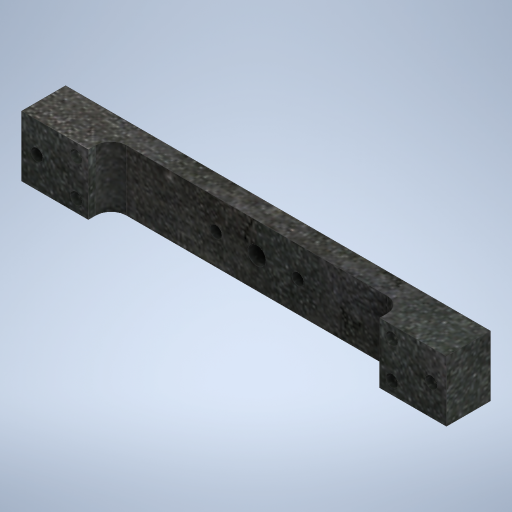
# Autodesk Inventor part: Uchwyt na ramę
Saved by Autodesk Inventor 2024 (Build 280153000, 153)
## iProperties
Created: 2024-04-14
Part Number: Uchwyt na ramę
Material: Steel
Document SubType Name: Sheet Metal
Designer: HP
Density: 7.85 g/cm^3
Sheet Metal Rule: Default
Appearance: Plate
Author: HP
Autodesk Inventor part; units mm, degrees
ref_plane "YZ Plane" through (0, 0, 0) normal (1, 0, 0) x (0, 1, 0)
ref_plane "XZ Plane" through (0, 0, 0) normal (0, 1, 0) x (-1, 0, 0)
ref_plane "XY Plane" through (0, 0, 0) normal (0, 0, 1) x (1, 0, 0)
sketch "Sketch1" plane through (0, 0, 0) normal (0, 0, 1) x (1, 0, 0)
  line L0 (-70, 10) -> (70, 10)
  line L1 (70, 10) -> (70, -10)
  line L2 (70, -10) -> (-70, -10)
  line L3 (-70, -10) -> (-70, 10)
  line L4 (-70, 10) -> (70, -10) construction
  line L5 (70, 10) -> (-70, -10) construction
  line L6 (0, 0) -> (-13.5, 0) construction
  line L7 (-13.5, 0) -> (13.5, 0) construction
  circle A0 centre (-13.5, 0) radius 2
  circle A1 centre (13.5, 0) radius 2
  circle A2 centre (0, 0) radius 3
  dimension "d0" = 140
  dimension "d1" = 20
  dimension "d2" = 13.5
  dimension "d3" = 27
  dimension "d4" = 4
  dimension "d5" = 4
  dimension "d6" = 6
  constraints: 16 end point, 3 centre point, 3 coincident, 2 horizontal, 2 midpoint, 2 parallel, 1 perpendicular, 1 point on line
  measures "d0" distance of L1.end L2.end
  measures "d1" distance of L0.end L1.end
  measures "d2" distance of L6.start L6.end
  measures "d3" distance of L6.end L7.end
  measures "d4" diameter of A0
  measures "d5" diameter of A1
  measures "d6" diameter of A2
extrude "Extrusion1" add sketch "Sketch1" along normal mid plane 7
sketch "Sketch2" plane through (-70, -10, 3.5) normal (0, -1, 0) x (1, 0, 0)
  line L0 (70, -3.5) -> (30, -3.5) construction
  line L1 (30, -3.5) -> (110, -3.5) construction
  line L2 (0, 0) -> (140, 0) projected
  line L3 (22, 5) -> (22, 7.5)
  line L4 (22, 7.5) -> (2, 7.5)
  line L5 (0, 5.5) -> (0, 0)
  line L6 (0, 0) -> (22, 0)
  line L7 (70, -9.525) -> (70, 0) construction
  line L8 (27, 0) -> (140, 0)
  arc A0 (22, 5) -> (27, 0) centre (27, 5) ccw
  line L9 (27, 0) -> (22, 0)
  line L10 (140, 0) -> (0, 0)
  line L11 (118, 5) -> (118, 7.5)
  line L12 (118, 7.5) -> (138, 7.5)
  line L13 (140, 5.5) -> (140, 0)
  arc A1 (113, 0) -> (118, 5) centre (113, 5) ccw
  line L14 (140, 5.5) -> (140, 7.5)
  line L15 (140, 7.5) -> (138, 7.5)
  line L16 (0, 5.5) -> (0, 7.5)
  line L17 (0, 7.5) -> (2, 7.5)
  point P0 (113, 0)
  dimension "d13" = 40
  dimension "d14" = 80
  dimension "d15" = 7.5
  dimension "d16" = 5
  constraints: 34 end point, 8 symmetric about line, 5 perpendicular, 4 point on circle, 4 point on line, 3 tangent, 2 centre point, 2 collinear, 2 horizontal, 2 vertical, 1 midpoint, 1 other
  measures "d13" distance of L0.start L0.end
  measures "d14" distance of L0.end L1.end
  measures "d15" distance of L6.end L3.end
  measures "d16" radius of A0
extrude "Extrusion2" add sketch "Sketch2" against normal blind 20
sketch "Sketch3" plane through (48, -10, 11) normal (0, 0, 1) x (1, 0, 0)
  line L0 (-48, 10) -> (12, 10) construction
  line L1 (12, 10) -> (17, 10) construction
  circle A0 centre (17, 10) radius 2
  line L2 (12, 10) -> (4, 10) construction
  line L3 (4, 10) -> (4, 4) construction
  line L4 (4, 4) -> (4, 16) construction
  circle A1 centre (4, 4) radius 2
  circle A2 centre (4, 16) radius 2
  line L5 (-48, 10) -> (-48, 19.9246) construction
  circle A3 centre (-113, 10) radius 2
  circle A4 centre (-100, 4) radius 2
  circle A5 centre (-100, 16) radius 2
  dimension "d20" = 60
  dimension "d21" = 5
  dimension "d22" = 4
  dimension "d23" = 8
  dimension "d24" = 6
  dimension "d25" = 12
  dimension "d26" = 4
  dimension "d27" = 4
  constraints: 12 end point, 6 centre point, 3 coincident, 3 point on line, 3 symmetric about line, 1 horizontal, 1 perpendicular, 1 vertical, 3 other
  measures "d20" distance of L0.start L0.end
  measures "d21" distance of L0.end L1.end
  measures "d22" diameter of A0
  measures "d23" distance of L0.end L2.end
  measures "d24" distance of L2.end L3.end
  measures "d25" distance of L3.end L4.end
  measures "d26" diameter of A1
  measures "d27" diameter of A2
extrude "Extrusion3" cut sketch "Sketch3" against normal blind 17.5
equation "\"BendRadius\" = Thickness"
equation "\"BendReliefWidth\" = Thickness"
equation "\"BendReliefDepth\" = 0.5 * Thickness"
equation "\"CornerReliefSize\" = 4 * Thickness"
equation "\"MinimumRemnant\" = 2 * Thickness"
equation "\"TransitionRadius\" = BendRadius"
equation "\"JacobiRadiusSize\" = BendRadius"
equation "\"GapSize\" = Thickness"
equation "\"Thickness\" = 3.048"
body "Solid1"
